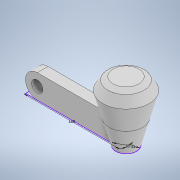
# Autodesk Inventor part: handle
Saved by Autodesk Inventor 2021 (Build 250183000, 183)
## iProperties
Created: 2021-03-11
Part Number: handle
Material: Generic
Document SubType Name: Modeling
Designer: ben
Density: 1 g/cm^3
Appearance: Default
Author: ben
Autodesk Inventor part; units mm, degrees
ref_plane "YZ Plane" through (0, 0, 0) normal (1, 0, 0) x (0, 1, 0)
ref_plane "XZ Plane" through (0, 0, 0) normal (0, 1, 0) x (-1, 0, 0)
ref_plane "XY Plane" through (0, 0, 0) normal (0, 0, 1) x (1, 0, 0)
sketch "Sketch1" plane through (0, 0, 0) normal (0, 0, 1) x (1, 0, 0)
  line L0 (25, -9) -> (-135, -9)
  line L1 (-135, -9) -> (-135, 9)
  line L2 (-135, 9) -> (25, 9)
  line L3 (25, 9) -> (25, -9)
  circle A0 centre (-135, 0) radius 17.5
  point P0 (0, 0)
  dimension "d0" = 160
  dimension "d1" = 18
  dimension "d5" = 35
  constraints: 8 end point, 2 parallel, 1 centre point, 1 horizontal, 1 midpoint, 1 perpendicular
  measures "d0" distance of L1.end L2.end
  measures "d1" distance of L0.end L1.end
  measures "d5" diameter of A0
extrude "Extrusion1" add sketch "Sketch1" along normal blind 40 contours L0 A0 L2 L3 | L0 L1 L2 A0 picked at (-129.1667, 0)
fillet "Fillet1" radius 20 2 edges at (25, 0, 40) (25, 0, 0)
extrude "Extrusion2" add sketch "Sketch1" along normal blind 40 draft 15 contours A0 L2 L1 L0 | L0 L1 L2 A0
sketch "Sketch4" plane through (0, 0, 40) normal (0, 0, 1) x (1, 0, 0)
  line L0 (-108.2558, -9) -> (5, -9) projected
  line L1 (5, 9) -> (5, -9) projected
  line L2 (5, 9) -> (-108.2558, 9) projected
  arc A0 (-108.2558, 9) -> (-108.2558, -9) centre (-135, 0) ccw projected
  circle A1 centre (-135, 0) radius 28.218
  point P0 (0, 0)
  constraints: 1 centre point, 1 coincident, 1 concentric
extrude "Extrusion3" add sketch "Sketch4" along normal blind 40 draft 15 separate body contours A0 A1
sketch "Sketch5" plane through (-135, 0, 80) normal (0, 0, 1) x (1, 0, 0)
  circle A0 centre (0, 0) radius 38.9359 projected
  point P0 (135, 0)
extrude "Extrusion4" add sketch "Sketch5" along normal blind 15 draft -30 bodies 2
sketch "Sketch6" plane through (-135, 0, 95) normal (0, 0, 1) x (1, 0, 0)
  circle A0 centre (0, 0) radius 30.2757 projected
  point P0 (135, 0)
extrude "Extrusion5" add sketch "Sketch6" along normal blind 5 draft -60 separate body
sketch "Sketch9" plane through (5, 9, 20) normal (0, 1, 0) x (1, 0, 0)
  circle A0 centre (0, 0) radius 9.525
  point P0 (-5, 20)
  dimension "d21" = 19.05
  constraints: 1 centre point
  measures "d21" diameter of A0
extrude "Extrusion8" cut sketch "Sketch9" against normal through all bodies 1
sketch "Sketch11" plane through (0, 0, 40) normal (0, 0, 1) x (1, 0, 0)
  arc A0 (-108.2558, 9) -> (-108.2558, -9) centre (-135, 0) ccw projected
  circle A1 centre (-135, 0) radius 10
  point P0 (0, 0)
  dimension "d27" = 20
  constraints: 1 centre point, 1 coincident
  measures "d27" diameter of A1
extrude "Extrusion10" add sketch "Sketch11" along normal blind 50 bodies 1
sketch "Sketch12" plane through (-135, 0, 95) normal (0, 0, -1) x (-1, 0, 0)
  circle A0 centre (0, 0) radius 10 projected
  point P0 (-135, 0)
extrude "Extrusion11" add sketch "Sketch12" along normal up to surface (5 mm away) bodies 3
sketch "Sketch13" plane through (-135, 0, 95) normal (0, 0, 1) x (1, 0, 0)
  circle A0 centre (0, 0) radius 10 projected
  point P0 (135, 0)
extrude "Extrusion12" cut sketch "Sketch13" against normal through all bodies 2
